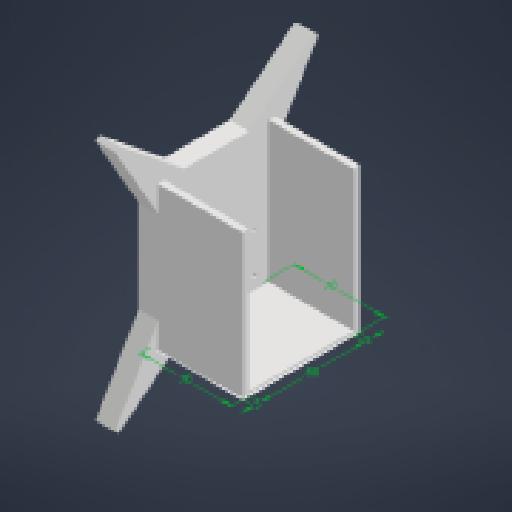
# Autodesk Inventor part: Part13
Saved by Autodesk Inventor 2027 (Build 310192060, 192F)
## iProperties
Created: 2026-08-17
Part Number: Part13
Material: Generic
Document SubType Name: Modeling
Designer: trtrn
Density: 1 g/cm^3
Appearance: Default
Author: trtrn
Autodesk Inventor part; units mm, degrees
ref_plane "YZ Plane" through (0, 0, 0) normal (1, 0, 0) x (0, 1, 0)
ref_plane "XZ Plane" through (0, 0, 0) normal (0, 1, 0) x (-1, 0, 0)
ref_plane "XY Plane" through (0, 0, 0) normal (0, 0, 1) x (1, 0, 0)
sketch "Sketch1" plane through (0, 0, 0) normal (0, 1, 0) x (-1, 0, 0)
  line L0 (35, 40) -> (-35, 40)
  line L1 (-35, 40) -> (-35, -40)
  line L2 (-35, -40) -> (35, -40)
  line L3 (35, -40) -> (35, 40)
  line L4 (35, 40) -> (-35, -40) construction
  line L5 (-35, 40) -> (35, -40) construction
  line L6 (35, 40) -> (-35, 40)
  line L7 (-35, 40) -> (-35, 45)
  line L8 (-35, 45) -> (35, 45)
  line L9 (35, 45) -> (35, 40)
  line L10 (35, -40) -> (-35, -40)
  line L11 (-35, -40) -> (-35, -45)
  line L12 (-35, -45) -> (35, -45)
  line L13 (35, -45) -> (35, -40)
  point P0 (0, 0)
  point P1 (-35, 40)
  dimension "d0" = 80
  dimension "d1" = 70
  dimension "d2" = 70
  dimension "d3" = 5
  dimension "d4" = 5
  constraints: 28 end point, 6 parallel, 3 horizontal, 3 perpendicular, 2 midpoint, 1 point on line
  measures "d0" distance of L1.end L0.end
  measures "d1" distance between parallel lines of L1 L3
  measures "d2" distance of L7.end L8.end
  measures "d3" distance of L6.end L7.end
  measures "d4" distance of L11.end L10.end
extrude "Extrusion1" add sketch "Sketch1" along normal blind 3 contours L3 L2 L1 L0
ref_plane "Work Plane1" through (198.5893, 154, -40.7) normal (0, 1, 0) x (0, 0, 1)
extrude "Extrusion2" add sketch "Sketch1" along normal up to surface (154 mm away) contours L0 L7 L8 L9 | L13 L12 L11 L2
sketch "Sketch8" plane through (-35, 3, -40) normal (0, 0, 1) x (1, 0, 0)
  line L0 (0, 0) -> (0, 151) projected
  line L1 (70, 0) -> (0, 0) projected
  line L2 (0, 0) -> (5, 0)
  line L3 (5, 0) -> (5, 151)
  line L4 (5, 151) -> (0, 151)
  line L5 (0, 151) -> (0, 0)
  line L6 (70, 151) -> (0, 151) projected
  point P0 (35, -3)
  point P1 (0, 151)
  dimension "d35" = 5
  constraints: 8 end point, 2 parallel, 1 collinear, 1 horizontal, 1 perpendicular
  measures "d35" distance of L4.end L3.end
extrude "Extrusion7" add sketch "Sketch8" along normal up to surface (80 mm away)
sketch "Sketch9" plane through (-35, 0, -45) normal (-1, 0, 0) x (0, 0, 1)
  circle A0 centre (16, 42.5) radius 1.65
  circle A1 centre (16, 12.5) radius 1.65
  circle A2 centre (74, 42.5) radius 1.65
  circle A3 centre (74, 12.5) radius 1.65
  point P0 (45, 0)
  constraints: 4 centre point, 8 other
extrude "Extrusion8" cut sketch "Sketch9" against normal blind 10
sketch "Sketch13" plane through (-35, 0, -45) normal (-1, 0, 0) x (0, 0, 1)
  line L0 (0, 0) -> (90, 0)
  line L1 (90, 0) -> (90, 154)
  line L2 (0, 154) -> (0, 0)
  line L3 (90, 0) -> (90, 154) projected
  line L4 (5, 5) -> (85, 5)
  line L5 (85, 5) -> (85, 149)
  line L6 (85, 149) -> (5, 149)
  line L7 (5, 149) -> (5, 5)
  line L8 (0, 154) -> (90, 154)
  line L9 (0, 0) -> (0, 154) projected
  line L10 (90, 154) -> (0, 154) projected
  point P0 (45, 0)
  dimension "d57" = 5
  dimension "d67" = 5
  dimension "d68" = 5
  constraints: 16 end point, 3 parallel, 3 perpendicular, 2 collinear, 1 horizontal, 1 other
  measures "d57" distance between parallel lines of L2 L7
  measures "d67" distance between parallel lines of L8 L6
  measures "d68" distance between parallel lines of L1 L5
extrude "Extrusion12" add sketch "Sketch13" along normal blind 10
sketch "Sketch14" plane through (-45, 0, -45) normal (-1, 0, 0) x (0, 0, 1)
  line L0 (0, 0) -> (90, 0) projected
  line L1 (0, 154) -> (0, 0) projected
  line L2 (90, 0) -> (90, 154) projected
  line L3 (45, 0) -> (45, 110.75) construction
  line L4 (90, 77) -> (0, 77) construction
  line L5 (-25.2284, -43.1686) -> (115.2284, 197.1686) construction
  line L6 (115.2284, -43.1686) -> (-25.2284, 197.1686) construction
  line L7 (116.9551, -42.1595) -> (113.5017, -44.1777)
  line L8 (70, 0) -> (113.5017, -44.1777)
  line L9 (90, 20) -> (116.9551, -42.1595)
  line L10 (90, 20) -> (90, 0)
  line L11 (70, 0) -> (90, 0)
  line L12 (-26.9551, -42.1595) -> (-23.5017, -44.1777)
  line L13 (20, 0) -> (-23.5017, -44.1777)
  line L14 (0, 20) -> (-26.9551, -42.1595)
  line L15 (116.9551, 196.1595) -> (113.5017, 198.1777)
  line L16 (70, 154) -> (113.5017, 198.1777)
  line L17 (90, 134) -> (116.9551, 196.1595)
  line L18 (0, 134) -> (-26.9551, 196.1595)
  line L19 (20, 154) -> (-23.5017, 198.1777)
  line L20 (-26.9551, 196.1595) -> (-23.5017, 198.1777)
  line L21 (90, 154) -> (0, 154) projected
  point P0 (45, 77)
  point P1 (90, 134)
  point P2 (0, 134)
  dimension "d61" = 20
  dimension "d62" = 20
  dimension "d63" = 50
  dimension "d64" = 4
  constraints: 36 end point, 14 symmetric about line, 5 midpoint, 4 point on line, 2 perpendicular, 1 vertical
  measures "d61" distance of L0.end L8.start
  measures "d62" distance of L0.end L9.start
  measures "d63" distance of L5.end L2.end
  measures "d64" distance of L7.start L7.end
extrude "Extrusion13" add sketch "Sketch14" against normal up to surface (15 mm away) contours L0 L13 L12 L14 L1 | L0 L2 L9 L7 L8 | L18 L20 L19 L21 L1 | L2 L21 L16 L15 L17
ref_plane "Work Plane2" through (277.5893, 154, 25) normal (0, 1, 0) x (1, 0, 0)
sketch "Sketch17" plane through (35, 0, 45) normal (1, 0, 0) x (0, 0, -1)
  line L0 (90, 0) -> (90, 154) projected
  line L1 (0, 0) -> (90, 0) projected
  line L2 (0, 0) -> (0, 154) projected
  line L3 (5, 3) -> (5, 154) projected
  line L4 (5, 154) -> (0, 154) projected
  line L5 (90, 154) -> (85, 154) projected
  line L6 (85, 3) -> (85, 154) projected
  line L7 (5, 3) -> (85, 3) projected
  point P0 (45, 0)
body "Solid1"
